# Autodesk Inventor part: PIC16F1823-14PINTSSOP
Saved by Autodesk Inventor 2016 SP1 (Build 200210100, 210)
## iProperties
Created: 2015-11-19
Part Number: PIC16F1823-14PINTSSOP
Material: Generic
Document SubType Name: Modeling
Designer: PhillipD
Density: 1 g/cm^3
Appearance: TSSOP14, PIC16F1823-14PINTSSOP
Author: PhillipD
Autodesk Inventor part; units mm, degrees
ref_plane "YZ Plane" through (0, 0, 0) normal (1, 0, 0) x (0, 1, 0)
ref_plane "XZ Plane" through (0, 0, 0) normal (0, 1, 0) x (-1, 0, 0)
ref_plane "XY Plane" through (0, 0, 0) normal (0, 0, 1) x (1, 0, 0)
sketch "TSSOP14, PIC16F1823-14PINTSSOP_69" plane through (0, 0, 0) normal (0, 0, 1) x (1, 0, 0)
  line L0 (-2.5908, 3.121) -> (2.5908, 3.121)
  line L1 (2.5908, 3.121) -> (2.5908, -3.121)
  line L2 (2.5908, -3.121) -> (-2.5908, -3.121)
  line L3 (-2.5908, -3.121) -> (-2.5908, 3.121)
  constraints: 8 end point
extrude "Extrusion1" add sketch "TSSOP14, PIC16F1823-14PINTSSOP_69" along normal blind 1
body "Solid1"
